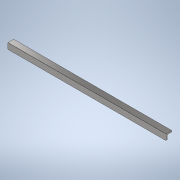
# Autodesk Inventor part: angulo_caja_calor
Saved by Autodesk Inventor 2021 (Build 250183000, 183)
## iProperties
Created: 2021-04-15
Part Number: angulo_caja_calor
Material: Acero inoxidable
Document SubType Name: Modeling
Designer: Leonardo Fabio Mercado Benítez
Density: 8 g/cm^3
Appearance: Semipulido
Author: Leonardo Fabio Mercado Benítez
Autodesk Inventor part; units mm, degrees
ref_plane "YZ Plane" through (0, 0, 0) normal (1, 0, 0) x (0, 1, 0)
ref_plane "XZ Plane" through (0, 0, 0) normal (0, 1, 0) x (-1, 0, 0)
ref_plane "XY Plane" through (0, 0, 0) normal (0, 0, 1) x (1, 0, 0)
sketch "Boceto1" plane through (0, 0, 0) normal (1, 0, 0) x (0, 1, 0)
  line L0 (0, -0.3) -> (0, -19.05)
  line L1 (-0.3, 0) -> (-19.05, 0)
  arc A0 (0, -0.3) -> (-0.3, 0) centre (-0.3, -0.3) ccw
  line L2 (-19.05, 0) -> (-19.05, -3.175)
  line L3 (0, -19.05) -> (-3.175, -19.05)
  line L4 (-3.175, -19.05) -> (-3.175, -3.475)
  line L5 (-3.475, -3.175) -> (-19.05, -3.175)
  arc A1 (-3.175, -3.475) -> (-3.475, -3.175) centre (-3.475, -3.475) ccw
  point P0 (0, 0)
  dimension "d0" = 19.05
  dimension "d1" = 19.05
  dimension "d2" = 0.3
  dimension "d3" = 3.175
  dimension "d4" = 3.175
  dimension "d5" = 0.3
  constraints: 12 end point, 4 point on circle, 4 tangent, 3 vertical, 2 centre point, 2 horizontal, 2 point on line, 1 perpendicular
  measures "d0" distance of point (0, 0) L0.end
  measures "d1" distance of point (0, 0) L1.end
  measures "d2" radius of A0
  measures "d3" distance of L1.end L2.end
  measures "d4" distance of L0.end L3.end
  measures "d5" radius of A1
extrude "Extrusión1" add sketch "Boceto1" along normal blind 515
fillet "Empalme1" radius 2 4 edges at (515, -19.05, -1.5875) (515, -1.5875, -19.05) (0, -19.05, -1.5875) (0, -1.5875, -19.05)
